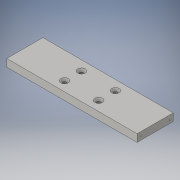
# Autodesk Inventor part: TopPlate
Saved by Autodesk Inventor 2016 (Build 200138000, 138)
## iProperties
Created: 2017-01-04
Part Number: TopPlate
Material: Generic
Document SubType Name: Modeling
Designer: james
Density: 1 g/cm^3
Appearance: Default
Author: james
Autodesk Inventor part; units mm, degrees
ref_plane "YZ Plane" through (0, 0, 0) normal (1, 0, 0) x (0, 1, 0)
ref_plane "XZ Plane" through (0, 0, 0) normal (0, 1, 0) x (-1, 0, 0)
ref_plane "XY Plane" through (0, 0, 0) normal (0, 0, 1) x (1, 0, 0)
sketch "Sketch1" plane through (0, 0, 0) normal (0, 1, 0) x (-1, 0, 0)
  line L0 (34.3448, 44.4205) -> (-185.3652, 44.4205)
  line L1 (-185.3652, 44.4205) -> (-185.3652, -16.5395)
  line L2 (-185.3652, -16.5395) -> (34.3448, -16.5395)
  line L3 (34.3448, -16.5395) -> (34.3448, 44.4205)
  point P0 (0, 0)
  dimension "d0" = 60.96
  dimension "d1" = 219.71
  constraints: 8 end point, 2 parallel, 1 horizontal, 1 perpendicular
  measures "d0" distance of L2.end L0.start
  measures "d1" distance of L1.end L2.end
extrude "Extrusion1" add sketch "Sketch1" along normal blind 12.7
sketch "Sketch2" plane through (0, 12.7, 0) normal (0, 1, 0) x (1, 0, 0)
  line L0 (-34.3448, -44.4205) -> (185.3652, -44.4205) projected
  line L1 (185.3652, 16.5395) -> (-34.3448, 16.5395) projected
  line L2 (-34.3448, 16.5395) -> (-34.3448, -44.4205) projected
  line L3 (185.3652, -44.4205) -> (185.3652, 16.5395) projected
  point P0 (0, 0)
  point P1 (46.9352, -28.1137)
  point P2 (46.9352, 0.2327)
  point P3 (104.2884, 0.2327)
  point P4 (104.2884, -28.1137)
  dimension "d4" = 28.3464
  dimension "d5" = 0
  dimension "d6" = 0
  dimension "d7" = 16.3068
  dimension "d8" = 16.3068
  dimension "d9" = 57.3532
  dimension "d10" = 0
  dimension "d11" = 0
  dimension "d12" = 81.28
  dimension "d13" = 81.0768
  measures "d4" distance of point (46.935, 0.233) point (46.935, -28.114)
  measures "d5" vertical distance of point (104.288, 0.233) point (46.935, 0.233)
  measures "d6" vertical distance of point (104.288, -28.114) point (46.935, -28.114)
  measures "d7" distance from line of L0 point (46.935, -28.114)
  measures "d8" distance from line of L1 point (46.935, 0.233)
  measures "d9" distance of point (104.288, -28.114) point (46.935, -28.114)
  measures "d10" horizontal distance of point (46.935, -28.114) point (46.935, 0.233)
  measures "d11" horizontal distance of point (104.288, -28.114) point (104.288, 0.233)
  measures "d12" distance from line of L2 point (46.935, -28.114)
  measures "d13" distance from line of L3 point (104.288, -28.114)
hole "Hole1" at (46.9352, 12.7, 28.1137) at (46.9352, 12.7, -0.2327) at (104.2884, 12.7, -0.2327) at (104.2884, 12.7, 28.1137) direction (0, -1, 0) diameter 6.35 end through all countersink diameter 12.7 countersink angle 82
sketch "Sketch5" plane through (-34.3448, 0, -16.5395) normal (-1, 0, 0) x (0, 0, 1)
  line L0 (0, 0) -> (0, 12.7) projected
  line L1 (0, 12.7) -> (60.96, 12.7) projected
  point P0 (16.5395, 0)
  point P1 (54.605, 5.7736)
  point P2 (6.35, 5.08)
  dimension "d21" = 48.26
  dimension "d22" = 6.35
  dimension "d23" = 7.62
  measures "d21" distance of point (6.35, 5.08) point (54.605, 5.774)
  measures "d22" distance from line of L0 point (6.35, 5.08)
  measures "d23" distance from line of L1 point (6.35, 5.08)
hole "Hole2" at (-34.3448, 5.7736, 38.0655) at (-34.3448, 5.08, -10.1895) direction (1, 0, 0) diameter 1.524 end through all
body "Solid1"
